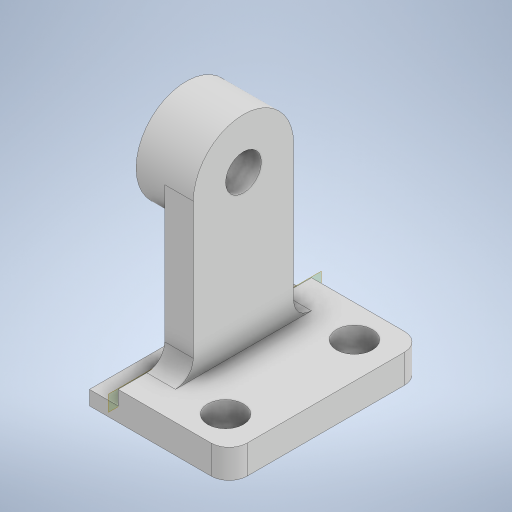
# Autodesk Inventor part: 4 - Part 1
Saved by Autodesk Inventor 2024 (Build 280153000, 153)
## iProperties
Created: 2024-04-20
Part Number: 4 - Part 1
Material: Generic
Document SubType Name: Modeling
Designer: Ricsi
Density: 1 g/cm^3
Appearance: Default
Author: Ricsi
Autodesk Inventor part; units mm, degrees
ref_plane "YZ Plane" through (0, 0, 0) normal (1, 0, 0) x (0, 1, 0)
ref_plane "XZ Plane" through (0, 0, 0) normal (0, 1, 0) x (-1, 0, 0)
ref_plane "XY Plane" through (0, 0, 0) normal (0, 0, 1) x (1, 0, 0)
sketch "Sketch1" plane through (0, 0, 0) normal (0, 1, 0) x (-1, 0, 0)
  line L0 (6.7034, 26.0749) -> (-27.2966, 26.0749)
  line L1 (-32.2966, 21.0749) -> (-32.2966, -22.9251)
  line L2 (-27.2966, -27.9251) -> (6.7034, -27.9251)
  line L3 (6.7034, -27.9251) -> (6.7034, 26.0749)
  arc A0 (-27.2966, 26.0749) -> (-32.2966, 21.0749) centre (-27.2966, 21.0749) ccw
  arc A1 (-32.2966, -22.9251) -> (-27.2966, -27.9251) centre (-27.2966, -22.9251) ccw
  circle A2 centre (-22.2966, 17.0749) radius 5
  circle A3 centre (-22.2966, -18.9251) radius 5
  point P0 (0, 0)
  point P1 (-32.2966, -27.9251)
  point P2 (-32.2966, 26.0749)
  dimension "d0" = 39
  dimension "d1" = 54
  dimension "d2" = 5
  dimension "d3" = 5
  dimension "d5" = 10
  dimension "d6" = 9
  dimension "d8" = 10
  dimension "d9" = 9
  constraints: 8 end point, 4 centre point, 4 point on circle, 4 point on line, 4 tangent, 2 parallel, 1 horizontal, 1 perpendicular
  measures "d0" distance of L2.end point (-32.297, -27.925)
  measures "d1" distance of point (-32.297, -27.925) point (-32.297, 26.075)
  measures "d2" radius of A0
  measures "d3" radius of A1
  measures "d5" diameter of A2
  measures "d6" distance from line of A2.centre L0
  measures "d8" diameter of A3
  measures "d9" distance from line of L2 A3.centre
extrude "Extrusion1" add sketch "Sketch1" along normal blind 8
sketch "Sketch2" plane through (0, 8, 0) normal (0, 1, 0) x (1, 0, 0)
  line L0 (-6.7034, 27.9251) -> (-6.7034, -26.0749) projected
  line L1 (-6.7034, -26.0749) -> (1.2966, -26.0749)
  line L2 (-6.7034, -26.0749) -> (27.2966, -26.0749) projected
  line L3 (1.2966, -26.0749) -> (1.2966, 27.9251)
  line L4 (1.2966, 27.9251) -> (-6.7034, 27.9251)
  line L5 (-6.7034, -26.0749) -> (-6.7034, 27.9251)
  point P0 (0, 0)
  dimension "d12" = 8
  dimension "d13" = 54
  constraints: 8 end point, 1 perpendicular, 1 point on line
  measures "d12" distance of L0.end L1.end
  measures "d13" distance of L1.end L3.end
extrude "Extrusion2" cut sketch "Sketch2" against normal blind 4
ref_plane "Work Plane2" through (1.2966, 8, -27.9251) normal (-1, 0, 0) x (0, 0, 1)
sketch "Sketch3" plane through (1.2966, 8, -27.9251) normal (-1, 0, 0) x (0, 0, 1)
  line L0 (0, 0) -> (54, 0) projected
  circle A0 centre (27, 43) radius 5
  arc A1 (41, 43) -> (13, 43) centre (27, 43) ccw
  line L1 (13, 43) -> (13, 0)
  line L2 (4, 0) -> (14, 0) projected
  line L3 (41, 43) -> (41, 0)
  line L4 (13, 0) -> (41, 0)
  point P0 (27.9251, -8)
  point P1 (13, 0)
  dimension "d19" = 10
  constraints: 6 end point, 2 centre point, 2 perpendicular, 2 point on circle, 2 point on line, 1 coincident, 1 collinear
  measures "d19" diameter of A0
extrude "Extrusion3" add sketch "Sketch3" against normal blind 8
fillet "Fillet1" radius 5 1 edges at (5.2966, 8, -14.9251)
fillet "Fillet2" radius 5 1 edges at (5.2966, 8, 13.0749)
sketch "Sketch4" plane through (1.2966, 4, -27.9251) normal (-1, 0, 0) x (0, 0, 1)
  line L0 (0, 0) -> (0, 4) projected
  circle A0 centre (27, 47) radius 14
  point P0 (27.9251, -4)
  constraints: 1 centre point
extrude "Extrusion4" add sketch "Sketch4" along normal blind 8
sketch "Sketch5" plane through (-6.7034, 51, -0.9251) normal (-1, 0, 0) x (0, 0, 1)
  circle A0 centre (0, 0) radius 5
  point P0 (0.9251, -51)
  dimension "d29" = 10
  constraints: 1 centre point
  measures "d29" diameter of A0
extrude "Extrusion5" cut sketch "Sketch5" against normal blind 8
body "Solid1"
